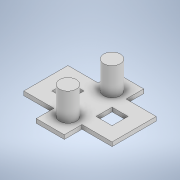
# Autodesk Inventor part: VexLegoWidget
Saved by Autodesk Inventor 2020 (Build 240168000, 168)
## iProperties
Created: 2020-02-28
Part Number: VexLegoWidget
Material: Generic
Document SubType Name: Modeling
Designer: Luke
Density: 1 g/cm^3
Appearance: Default
Author: Luke
Autodesk Inventor part; units mm, degrees
ref_plane "YZ Plane" through (0, 0, 0) normal (1, 0, 0) x (0, 1, 0)
ref_plane "XZ Plane" through (0, 0, 0) normal (0, 1, 0) x (-1, 0, 0)
ref_plane "XY Plane" through (0, 0, 0) normal (0, 0, 1) x (1, 0, 0)
sketch "Sketch7" plane through (0, 0, 0) normal (0, 1, 0) x (-1, 0, 0)
  line L0 (12.7, 6.35) -> (4.0386, 6.35)
  line L1 (-12.7, 6.35) -> (-12.7, -6.35)
  line L2 (-12.7, -6.35) -> (-4.0386, -6.35)
  line L3 (12.7, -6.35) -> (12.7, 6.35)
  line L4 (12.7, 6.35) -> (-12.7, -6.35) construction
  line L5 (-12.7, 6.35) -> (12.7, -6.35) construction
  line L6 (8.6614, 2.3114) -> (4.0386, 2.3114)
  line L7 (4.0386, 2.3114) -> (4.0386, -2.3114)
  line L8 (4.0386, -2.3114) -> (8.6614, -2.3114)
  line L9 (8.6614, -2.3114) -> (8.6614, 2.3114)
  line L10 (8.6614, 2.3114) -> (4.0386, -2.3114) construction
  line L11 (4.0386, 2.3114) -> (8.6614, -2.3114) construction
  line L12 (-8.6614, 2.3114) -> (-4.0386, 2.3114)
  line L13 (-4.0386, 2.3114) -> (-4.0386, -2.3114)
  line L14 (-4.0386, -2.3114) -> (-8.6614, -2.3114)
  line L15 (-8.6614, -2.3114) -> (-8.6614, 2.3114)
  line L16 (-8.6614, 2.3114) -> (-4.0386, -2.3114) construction
  line L17 (-4.0386, 2.3114) -> (-8.6614, -2.3114) construction
  line L18 (4.0386, 6.35) -> (4.0386, 11.43)
  line L19 (4.0386, 11.43) -> (-4.0386, 11.43)
  line L20 (-4.0386, 11.43) -> (-4.0386, 6.35)
  line L21 (-4.0386, -6.35) -> (-4.0386, -11.43)
  line L22 (-4.0386, -11.43) -> (4.0386, -11.43)
  line L23 (4.0386, -11.43) -> (4.0386, -6.35)
  line L24 (-4.0386, 6.35) -> (-12.7, 6.35)
  line L25 (4.0386, -6.35) -> (12.7, -6.35)
  point P0 (0, 0)
  point P1 (6.35, 0)
  point P2 (-6.35, 0)
  dimension "d29" = 25.4
  dimension "d30" = 12.7
  dimension "d31" = 4.6228
  dimension "d32" = 4.6228
  dimension "d33" = 4.6228
  dimension "d34" = 4.6228
  dimension "d35" = 12.7
  dimension "d36" = 6.35
  dimension "d37" = 5.08
  dimension "d40" = 5.08
  constraints: 52 end point, 9 parallel, 8 perpendicular, 6 midpoint, 4 horizontal, 4 point on line, 1 vertical
  measures "d29" distance of L3.start L1.end
  measures "d30" distance of L1.end L1.start
  measures "d31" distance of L8.end L7.end
  measures "d32" distance of L7.end L6.end
  measures "d33" distance of L13.end L14.end
  measures "d34" distance of L12.end L13.end
  measures "d35" distance of point (-6.35, 0) point (6.35, 0)
  measures "d36" distance of point (0, 0) point (6.35, 0)
  measures "d37" distance of L0.end L18.end
  measures "d40" distance of L22.end L23.end
extrude "Extrusion2" add sketch "Sketch7" along normal blind 1.1684
sketch "Sketch8" plane through (0, 1.1684, 0) normal (0, 1, 0) x (1, 0, 0)
  circle A0 centre (0, -6.35) radius 2.4003
  point P0 (0, 0)
  dimension "d47" = 4.8006
  dimension "d49" = 6.35
  constraints: 1 centre point
  measures "d47" diameter of A0
  measures "d49" distance of point (0, 0) A0.centre
sketch "Sketch9" plane through (0, 1.1684, 0) normal (0, 1, 0) x (1, 0, 0)
  circle A0 centre (0, 6.35) radius 2.4003
  point P0 (0, 0)
  dimension "d51" = 4.8006
  dimension "d52" = 6.35
  constraints: 1 centre point
  measures "d51" diameter of A0
  measures "d52" distance of point (0, 0) A0.centre
extrude "Extrusion3" add sketch "Sketch8" along normal blind 8.001
extrude "Extrusion4" add sketch "Sketch9" along normal blind 8.001
body "Solid3"
